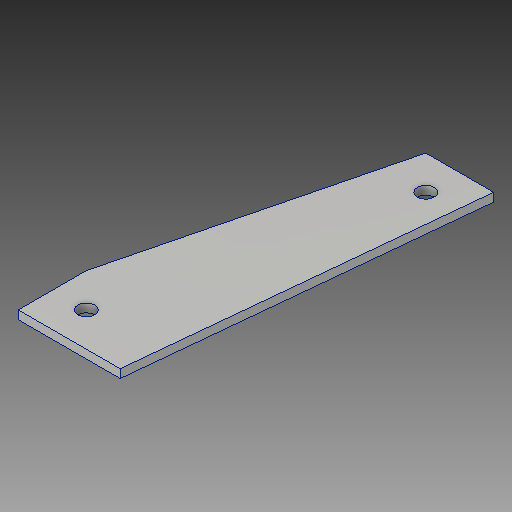
# Autodesk Inventor part: 15102898-16-P-0213
Saved by Autodesk Inventor 2017 (Build 210142000, 142)
## iProperties
Created: 2016-10-05
Part Number: 15102898-16-P-0213
Material: Aluminum 6061
Document SubType Name: Modeling
Designer: gus
Density: 2.7 g/cm^3
Appearance: Aluminum - Flat
Mass: 36.7888 g
Surface Area: 97.2966 cm^2
Volume: 13.6255 cm^3
Author: gus
Autodesk Inventor part; units mm, degrees
ref_plane "YZ Plane" through (0, 0, 0) normal (1, 0, 0) x (0, 1, 0)
ref_plane "XZ Plane" through (0, 0, 0) normal (0, 1, 0) x (-1, 0, 0)
ref_plane "XY Plane" through (0, 0, 0) normal (0, 0, 1) x (1, 0, 0)
sketch "Sketch1" plane through (0, 0, 0) normal (0, 1, 0) x (-1, 0, 0)
  line L0 (19.3231, -122.2306) -> (-6.0769, -122.2306)
  circle A0 centre (32.0231, -7.9306) radius 3.175
  circle A1 centre (6.6231, -109.5306) radius 3.175
  line L1 (19.3231, -122.2306) -> (44.7231, -20.6306)
  line L2 (44.7231, -20.6306) -> (44.7231, 4.7694)
  line L3 (-6.0769, -122.2306) -> (6.6231, 4.7694)
  line L4 (6.6231, 4.7694) -> (44.7231, 4.7694)
  dimension "d0" = 25.4
  dimension "d2" = 6.35
  dimension "d3" = 6.35
  dimension "d6" = 12.7
  dimension "d10" = 25.4
  dimension "d12" = 12.7
  dimension "d13" = 38.1
  dimension "d14" = 12.7
  dimension "d15" = 12.7
  dimension "d16" = 50.8
  dimension "d17" = 127
  constraints: 10 end point, 2 centre point, 1 horizontal, 1 parallel, 1 vertical
  measures "d0" distance of L0.start L0.end
  measures "d2" diameter of A0
  measures "d3" diameter of A1
  measures "d6" distance from line of L0 A1.centre
  measures "d10" distance of L1.end L2.end
  measures "d12" distance from line of L2 A0.centre
  measures "d13" distance of L3.end L2.end
  measures "d14" horizontal distance of L0.end A1.centre
  measures "d15" distance from line of L4 A0.centre
  measures "d16" horizontal distance of L0.end L2.end
  measures "d17" distance between parallel lines of L0 L4
extrude "Extrusion1" add sketch "Sketch1" along normal blind 3.175
body "Solid1"
